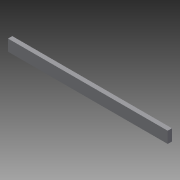
# Autodesk Inventor part: nd-p
Saved by Autodesk Inventor 2015 (Build 190159000, 159)
## iProperties
Created: 2014-07-02
Part Number: nd-p
Material: Generic
Document SubType Name: Modeling
Designer: peter
Density: 1 g/cm^3
Appearance: Default
Author: peter
Autodesk Inventor part; units mm, degrees
ref_plane "YZ Plane" through (0, 0, 0) normal (1, 0, 0) x (0, 1, 0)
ref_plane "XZ Plane" through (0, 0, 0) normal (0, 1, 0) x (-1, 0, 0)
ref_plane "XY Plane" through (0, 0, 0) normal (0, 0, 1) x (1, 0, 0)
sketch "Sketch1" plane through (0, 0, 0) normal (0, 0, 1) x (1, 0, 0)
  line L0 (711.1998, -0.1285) -> (254.0083, -0.1285)
  line L1 (254.0083, -0.1285) -> (-0.0002, -0.1285)
  line L2 (-0.0002, -0.1285) -> (-0.0002, 50.6715)
  line L3 (-0.0002, 50.6715) -> (254.0083, 50.6715)
  line L4 (254.0083, 50.6715) -> (711.1998, 50.6715)
  line L5 (711.1998, 50.6715) -> (711.1998, -0.1285)
  point P0 (0, 0)
  constraints: 12 end point
extrude "Extrusion1" add sketch "Sketch1" along normal blind 19.05
body "Solid1"
